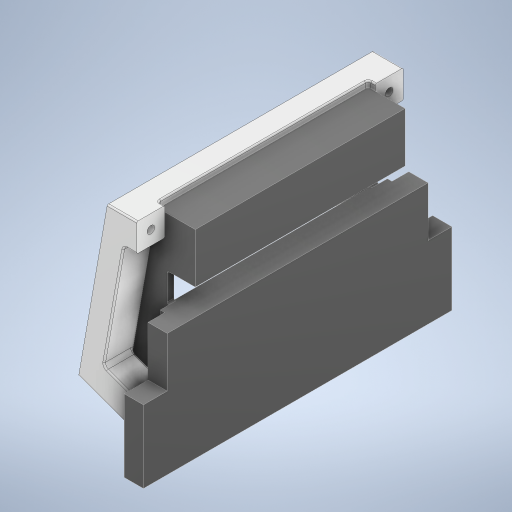
# Autodesk Inventor part: Display Cover
Saved by Autodesk Inventor 2024 (Build 280153000, 153)
## iProperties
Created: 2024-10-16
Part Number: Display Cover
Material: ABS Plastic
Document SubType Name: Modeling
Designer: Ishaan
Density: 1.06 g/cm^3
Appearance: Smooth - White
Author: Ishaan
Autodesk Inventor part; units mm, degrees
sketch "Sketch1" plane through (0, 0, 0) normal (0, 0, 1) x (1, 0, 0)
  line L0 (10.2452, 58.1037) -> (-10.2452, -58.1037)
  line L1 (-10.2452, -58.1037) -> (34.2452, -74.2969)
  line L2 (34.2452, -74.2969) -> (34.2452, -53.0133)
  line L3 (34.2452, -53.0133) -> (7.5941, -43.3131)
  line L4 (7.5941, -43.3131) -> (21.9501, 38.1037)
  line L5 (21.9501, 38.1037) -> (26.2452, 38.1037)
  line L6 (26.2452, 38.1037) -> (26.2452, 58.1037)
  line L7 (26.2452, 58.1037) -> (10.2452, 58.1037)
  point P0 (0, 0)
  point P1 (0, 0)
  dimension "d6" = 118
  dimension "d7" = 20
  dimension "d8" = 15
  dimension "d9" = 100
  dimension "d10" = 100
  dimension "d11" = 20
  dimension "d12" = 16
  dimension "d45" = 8
  constraints: 16 end point, 2 parallel, 2 perpendicular, 1 coincident, 1 horizontal, 1 midpoint, 1 vertical
  measures "d6" distance of L0.start L0.end
  measures "d7" distance of L5.end L6.end
  measures "d8" distance between parallel lines of L0 L4
  measures "d9" angle of L0 L7
  measures "d10" angle of L0 L1
  measures "d11" distance between parallel lines of L1 L3
  measures "d12" distance of L6.end L0.start
  measures "d45" distance between parallel lines of L6 L2
extrude "Extrusion1" add sketch "Sketch1" along normal mid plane 190
ref_plane "Work Plane1" through (1.5725, -60.1874, -95) normal (-0.9848078, 0.1736482, 0) x (0, 0, 1)
sketch "Sketch2" plane through (-10.2452, -58.1037, -95) normal (-0.9848078, 0.1736482, 0) x (0, 0, 1)
  line L0 (190, 0) -> (0, 0) projected
  line L1 (190, 118) -> (190, 0) projected
  line L2 (0, 118) -> (190, 118) projected
  line L3 (0, 0) -> (0, 118) projected
  line L4 (188, 116) -> (188, 2)
  line L5 (188, 2) -> (2, 2)
  line L6 (2, 2) -> (2, 116)
  line L7 (2, 116) -> (188, 116)
  point P0 (95, 59)
  dimension "d16" = 2
  constraints: 8 end point, 3 other
  measures "d16" distance between parallel lines of L2 L7
extrude "Extrusion2" cut sketch "Sketch2" against normal up to surface (12 mm away) contours L4 L5 L6 L7
sketch "Sketch3" plane through (26.2452, 38.1037, 95) normal (1, 0, 0) x (0, 0, -1)
  line L0 (190, 20) -> (0, 20) projected
  line L1 (0, 0) -> (0, 20) projected
  line L2 (190, 0) -> (0, 0) projected
  line L3 (190, 20) -> (190, 0) projected
  line L4 (0, 20) -> (20, 20)
  line L5 (20, 20) -> (20, 0)
  line L6 (20, 0) -> (0, 0)
  line L7 (0, 0) -> (0, 20)
  line L8 (190, 20) -> (170, 20)
  line L9 (170, 20) -> (170, 0)
  line L10 (170, 0) -> (190, 0)
  line L11 (190, 0) -> (190, 20)
  point P0 (95, -38.1037)
  point P1 (170, 20)
  point P2 (20, 20)
  dimension "d19" = 20
  dimension "d20" = 20
  constraints: 16 end point, 4 parallel, 2 horizontal, 2 perpendicular, 2 point on line
  measures "d19" distance of L5.end L6.end
  measures "d20" distance between parallel lines of L3 L9
extrude "Extrusion3" add sketch "Sketch3" along normal blind 5 contours L3 L2 L9 L0 | L5 L2 L1 L0
sketch "Sketch4" plane through (34.2452, -74.2969, -95) normal (-0.3420201, -0.9396926, 0) x (0.9396926, -0.3420201, 0)
  line L0 (0, 0) -> (0, 190) projected
  line L1 (-47.3458, 190) -> (0, 190) projected
  line L2 (-47.3458, 190) -> (-47.3458, 0) projected
  line L3 (0, 0) -> (-47.3458, 0) projected
  line L4 (0, 20) -> (-31.3458, 20)
  line L5 (-31.3458, 20) -> (-31.3458, 170)
  line L6 (-31.3458, 170) -> (0, 170)
  line L7 (0, 170) -> (0, 20)
  line L8 (-45.9608, 20) -> (-41.2623, 20) construction
  line L9 (-45.9608, 170) -> (-41.2623, 170) construction
  point P0 (-57.591, 95)
  point P1 (0, 170)
  dimension "d25" = 16
  constraints: 8 end point, 2 collinear, 2 parallel, 1 horizontal, 1 perpendicular, 1 point on line
  measures "d25" distance between parallel lines of L2 L5
extrude "Extrusion4" cut sketch "Sketch4" against normal blind 1 contours L4 L5 L6 L0
ref_plane "Work Plane2" through (34.2452, -74.2969, 95) normal (0.9396926, -0.3420201, 0) x (0.3420201, 0.9396926, 0)
sketch "Sketch9" plane through (0, 0, 0) normal (0, 0, 1) x (1, 0, 0)
  line L0 (21.7156, 54.0503) -> (9.8979, 56.134) projected
  line L1 (9.8979, 56.134) -> (10.2452, 58.1037) projected
  line L2 (10.2452, 58.1037) -> (26.2452, 58.1037) projected
  line L3 (26.2452, 58.1037) -> (26.2452, 38.1037) projected
  line L4 (26.2452, 38.1037) -> (21.9501, 38.1037) projected
  line L5 (21.9501, 38.1037) -> (7.5941, -43.3131) projected
  line L6 (34.2452, -53.0133) -> (34.2452, -73.2327) projected
  line L7 (34.2452, -73.2327) -> (5.1319, -62.6363) projected
  line L8 (5.1319, -62.6363) -> (4.7898, -63.576) projected
  line L9 (4.7898, -63.576) -> (-10.2452, -58.1037) projected
  line L10 (-10.2452, -58.1037) -> (-9.8979, -56.134) projected
  line L11 (-9.8979, -56.134) -> (1.9197, -58.2178) projected
  line L12 (1.9197, -58.2178) -> (21.7156, 54.0503) projected
  line L13 (21.9501, 38.1037) -> (18.9038, 38.1037)
  line L14 (7.5941, -43.3131) -> (30.2452, -51.5574) construction
  line L15 (21.7156, 54.0503) -> (1.9197, -58.2178) projected
  line L16 (7.5941, -43.3131) -> (34.2452, -53.0133) projected
  line L17 (1.9197, -58.2178) -> (12.9595, -60.1644)
  line L18 (12.9595, -60.1644) -> (34.2452, -67.9118)
  line L19 (7.5941, -43.3131) -> (4.8742, -58.7388)
  point P0 (0, 0)
  dimension "d54" = 5
  constraints: 8 end point, 3 point on line, 2 collinear, 1 horizontal, 1 parallel
  measures "d54" distance between parallel lines of L7 L18
extrude "Extrusion7" cut sketch "Sketch9" along normal mid plane 140 contours L13 L5 L19 L17 L12 | L19 L16 L6 L18 L17
extrude "Extrusion8" cut sketch "Sketch9" along normal up to surface (150 mm away) from surface at -75 contours L19 L16 L6 L18 L17
fillet "Fillet14" radius 1 2 edges at (13.4121, -10.3176, -70) (13.4121, -10.3176, 70)
fillet "Fillet9" radius 1 2 edges at (20.9197, -48.1632, 75) (20.9197, -48.1632, -75)
fillet "Fillet10" radius 3 8 edges at (7.5425, -43.606, -75.2929) (6.146, -51.5259, -75) (7.5941, -43.3131, -85.5) (7.5425, -43.606, 75.2929) (6.146, -51.5259, 75) (7.5941, -43.3131, 85.5) (21.9501, 38.1037, 83) (21.9501, 38.1037, -83)
fillet "Fillet11" radius 10 1 edges at (12.9595, -60.1644, 0)
fillet "Fillet12" radius 2 4 edges at (26.2452, 48.1037, 75) (26.2452, 48.1037, -75) (4.9612, -63.1052, -75) (4.9612, -63.1052, 75)
fillet "Fillet13" radius 1 28 edges at (26.2452, 38.1037, 0) (26.831, 38.1037, -74.4142) (29.7452, 38.1037, -75) (29.7452, 38.1037, 75) (26.831, 38.1037, 74.4142) (26.831, 58.1037, 74.4142) (29.7452, 58.1037, 75) (26.831, 58.1037, -74.4142) (29.7452, 58.1037, -75) (26.2452, 58.1037, 0) (20.7452, 58.1037, -95) (20.7452, 58.1037, 95) (8.3876, -42.855, 95) (14.7721, -2.6047, 95) (27.8563, 38.1037, 95) (22.1024, -48.5937, 95) (8.3876, -42.855, -95) (22.1024, -48.5937, -95) (22.539, 37.4018, -95) (27.8563, 38.1037, -95) (14.7721, -2.6047, -95) (12, -66.2003, -95) (5.3403, -63.7763, -74.4142) (4.7898, -63.576, 0) (5.3403, -63.7763, 74.4142) (20.4572, -69.2784, 75) (20.4572, -69.2784, -75) (12, -66.2003, 95)
fillet "Fillet16" radius 1 3 edges at (10.1473, -11.5571, -70) (18.9038, 38.1037, 0) (10.1473, -11.5571, 70)
sketch "Sketch12" plane through (31.2452, 38.1037, 95) normal (1, 0, 0) x (0, 0, -1)
  line L0 (19, 20) -> (1, 20) projected
  line L1 (189, 20) -> (171, 20) projected
  line L2 (190, 1) -> (190, 19) projected
  point P0 (95, -38.1037)
  point P1 (10, 10)
  point P2 (180, 10)
  point P3 (10, 20)
  point P4 (180, 20)
  point P5 (190, 10)
  constraints: 3 midpoint, 2 horizontal alignment, 2 vertical alignment
hole "Hole4" at (31.2452, 48.1037, 85) at (31.2452, 48.1037, -85) direction (-1, 0, 0) diameter 5.4 end through all
ref_plane "Work Plane3" through (26.2452, 38.1037, 95) normal (1, 0, 0) x (0, 0, -1)
sketch "Sketch13" plane through (26.2452, 38.1037, 95) normal (1, 0, 0) x (0, 0, -1)
  circle A0 centre (10, 10) radius 2.7 projected
  circle A1 centre (10, 10) radius 2.7 projected
  circle A2 centre (180, 10) radius 2.7 projected
  circle A3 centre (180, 10) radius 2.7 projected
  point P0 (95, -38.1037)
hole "Hole5" at (26.2452, 48.1037, -85) at (26.2452, 48.1037, 85) direction (-1, 0, 0) diameter 9.5 end through all
sketch "Sketch14" plane through (0, 0, 0) normal (0, 0, 1) x (1, 0, 0)
  line L0 (9.8979, 56.134) -> (10.2452, 58.1037) projected
  line L1 (10.2452, 58.1037) -> (25.2452, 58.1037) projected
  arc A0 (26.2452, 57.1037) -> (25.2452, 58.1037) centre (25.2452, 57.1037) ccw projected
  line L2 (26.2452, 57.1037) -> (26.2452, 39.1037) projected
  arc A1 (25.2452, 38.1037) -> (26.2452, 39.1037) centre (25.2452, 39.1037) ccw projected
  line L3 (25.2452, 38.1037) -> (20.0956, 38.1037) projected
  arc A2 (19.1108, 39.2773) -> (20.0956, 38.1037) centre (20.0956, 39.1037) ccw projected
  line L4 (19.1108, 39.2773) -> (21.7156, 54.0503) projected
  line L5 (21.7156, 54.0503) -> (9.8979, 56.134) projected
  arc A3 (13.7816, -60.4637) -> (12.0979, -60.0125) centre (10.3614, -69.8606) ccw projected
  line L6 (13.7816, -60.4637) -> (34.2452, -67.9118) projected
  line L7 (34.2452, -67.9118) -> (34.2452, -73.2327) projected
  line L8 (34.2452, -73.2327) -> (5.1319, -62.6363) projected
  arc A4 (3.8501, -63.234) -> (5.1319, -62.6363) centre (4.1922, -62.2943) ccw projected
  line L9 (3.8501, -63.234) -> (-10.2452, -58.1037) projected
  line L10 (-10.2452, -58.1037) -> (-9.8979, -56.134) projected
  line L11 (-9.8979, -56.134) -> (12.0979, -60.0125) projected
  line L12 (52.9452, -1.8963) -> (32.9452, -1.8963) construction
  line L13 (32.9452, -1.8963) -> (32.9452, 18.1037) construction
  line L14 (32.9452, 18.1037) -> (52.9452, 18.1037) construction
  line L15 (52.9452, 18.1037) -> (52.9452, -1.8963) construction
  line L16 (52.9452, -1.8963) -> (32.9452, 18.1037) construction
  line L17 (32.9452, -1.8963) -> (52.9452, 18.1037) construction
  line L18 (52.9452, -1.8963) -> (72.9452, -1.8963) construction
  line L19 (72.9452, -1.8963) -> (72.9452, 53.8537) construction
  line L20 (72.9452, 53.8537) -> (52.9452, 53.8537) construction
  line L21 (52.9452, 53.8537) -> (52.9452, -1.8963) construction
  line L22 (31.2452, 58.1037) -> (28.2452, 58.1037) construction
  line L23 (31.2452, 57.1037) -> (31.2452, 39.1037) construction
  line L24 (52.7452, 53.8537) -> (52.7452, 18.3037)
  line L25 (52.7452, 18.3037) -> (32.7452, 18.3037)
  line L26 (32.7452, -2.0963) -> (50.9452, -2.0963)
  line L27 (50.9452, -2.0963) -> (50.9452, -89.3802)
  line L28 (50.9452, -89.3802) -> (33.9452, -89.3802)
  line L29 (33.9452, -89.3802) -> (33.9452, -52.4785)
  line L30 (33.9452, -52.4785) -> (8.0463, -43.052)
  line L31 (8.0463, -43.052) -> (22.2857, 37.7037)
  line L32 (22.2857, 37.7037) -> (26.6452, 37.7037)
  line L33 (26.6452, 37.7037) -> (26.6452, 53.8537)
  line L34 (26.6452, 53.8537) -> (52.7452, 53.8537)
  line L35 (32.7452, 18.3037) -> (32.7452, -2.0963)
  line L36 (34.2452, -53.0133) -> (9.9596, -44.1741) projected
  arc A5 (8.0313, -40.834) -> (9.9596, -44.1741) centre (10.9857, -41.355) ccw projected
  line L37 (4.8742, -58.7388) -> (21.513, 35.6246) projected
  circle A6 centre (10.9857, -41.355) radius 2.6
  line L38 (28.2452, 38.1037) -> (31.2452, 38.1037) projected
  arc A7 (24.4674, 38.1037) -> (21.513, 35.6246) centre (24.4674, 35.1037) ccw projected
  circle A8 centre (24.4674, 35.1037) radius 2.6
  line L39 (26.6452, 37.7037) -> (52.7452, 37.7037)
  line L40 (33.9452, -89.3802) -> (37.1952, -89.3802)
  line L41 (37.1952, -89.3802) -> (37.1952, -77.3802)
  line L42 (37.1952, -77.3802) -> (33.9452, -77.3802)
  line L43 (33.9452, -77.3802) -> (33.9452, -89.3802)
  line L44 (-10.2452, -58.1037) -> (34.2452, -74.2969) construction
  line L45 (33.9452, -77.3802) -> (23.2544, -73.4891) construction
  line L46 (33.9452, -67.3769) -> (5.5778, -57.052)
  line L47 (5.5778, -57.052) -> (8.0463, -43.052)
  line L48 (33.9452, -52.4785) -> (47.9452, -57.574)
  line L49 (47.9452, -57.574) -> (47.9452, 37.7037)
  line L50 (32.7452, -2.0963) -> (47.9452, -2.0963)
  line L51 (47.9452, -2.0963) -> (47.9452, -9.0963)
  line L52 (47.9452, -9.0963) -> (32.7452, -9.0963)
  line L53 (32.7452, -9.0963) -> (32.7452, -2.0963)
  line L54 (33.9452, -67.3769) -> (47.9452, -72.4725)
  line L55 (47.9452, -72.4725) -> (47.9452, -57.574)
  point P0 (0, 0)
  point P1 (42.9452, 8.1037)
  point P2 (24.4674, 37.7037)
  point P3 (21.9069, 35.5551)
  point P4 (8.4252, -40.9035)
  point P5 (10.0964, -43.7982)
  point P6 (10.0964, -43.7982)
  point P7 (47.9452, 18.3037)
  dimension "d98" = 20
  dimension "d99" = 20
  dimension "d100" = 4.25
  dimension "d101" = 45.75
  dimension "d102" = 20
  dimension "d104" = 21.7
  dimension "d105" = 32.9452
  dimension "d106" = 0.2
  dimension "d107" = 0.4
  dimension "d108" = 0.2
  dimension "d109" = 0.2
  dimension "d110" = 1
  dimension "d111" = 0.2
  dimension "d112" = 0.4
  dimension "d113" = 0.4
  dimension "d114" = 0.4
  dimension "d115" = 8
  dimension "d116" = 3.25
  dimension "d117" = 12
  dimension "d118" = 3
  dimension "d142" = 0.4
  dimension "d146" = 3
  dimension "d147" = 7
  constraints: 76 end point, 14 parallel, 10 perpendicular, 5 collinear, 4 horizontal, 4 point on line, 2 centre point, 2 coincident, 2 midpoint, 2 tangent, 1 vertical
  measures "d98" distance of L13.end L14.end
  measures "d99" distance of L12.end L13.end
  measures "d100" distance between parallel lines of L20 L22
  measures "d101" distance from line of L20 point (42.945, 8.104)
  measures "d102" distance between parallel lines of L19 L21
  measures "d104" distance between parallel lines of L21 L23
  measures "d105" distance from line of point (0, 0) L13
  measures "d106" distance between parallel lines of L21 L24
  measures "d107" distance between parallel lines of L33 L2
  measures "d108" distance between parallel lines of L25 L14
  measures "d109" distance between parallel lines of L12 L26
  measures "d110" distance between parallel lines of L29 L13
  measures "d111" distance between parallel lines of L13 L35
  measures "d112" distance between parallel lines of L30 L36
  measures "d113" distance between parallel lines of L37 L31
  measures "d114" distance between parallel lines of L38 L32
  measures "d115" distance from line of L27 point (42.945, 8.104)
  measures "d116" distance between parallel lines of L29 L41
  measures "d117" distance of L40.end L41.end
  measures "d118" distance between parallel lines of L44 L45
  measures "d142" distance between parallel lines of L46 L6
  measures "d146" distance between parallel lines of L27 L49
  measures "d147" distance between parallel lines of L26 L52
ref_plane "Work Plane4" through (0, 0, 98) normal (0, 0, 1) x (1, 0, 0)
ref_plane "Work Plane5" through (0, 0, -98) normal (0, 0, -1) x (-1, 0, 0)
extrude "Extrusion9" add sketch "Sketch14" along normal up to surface (196 mm away) from surface at -98 separate body contours L29 L54 L55 L49 L26 L27 L28 L41 L42 L8 L7 L6 | L6 L7 L8 L29 | L29 L48 L55 L54 | L30 A6 L31 A8 L32 L39 L49 L25 L35 L53 L52 L48 | A6 | L52 L53 L26 L49 | A8 | L49 L39 L24 L25
sketch "Sketch15" plane through (24.4674, 37.7037, 98) normal (0, 1, 0) x (1, 0, 0)
  line L0 (6.7778, 23) -> (3.7778, 23) projected
  arc A0 (1.7778, 25) -> (3.7778, 23) centre (3.7778, 25) ccw projected
  line L1 (1.7778, 25) -> (1.7778, 171) projected
  arc A1 (3.7778, 173) -> (1.7778, 171) centre (3.7778, 171) ccw projected
  line L2 (3.7778, 173) -> (6.7778, 173) projected
  line L3 (28.2778, 23.2) -> (3.7778, 23.2)
  arc A2 (1.9778, 25) -> (3.7778, 23.2) centre (3.7778, 25) ccw
  line L4 (1.9778, 25) -> (1.9778, 171)
  arc A3 (3.7778, 172.8) -> (1.9778, 171) centre (3.7778, 171) ccw
  line L5 (3.7778, 172.8) -> (28.2778, 172.8)
  line L6 (28.2778, 196) -> (28.2778, 0) projected
  point P0 (-24.4674, 98)
  dimension "d123" = 0.2
  constraints: 6 end point, 4 point on circle, 2 centre point, 2 point on line, 4 other
  measures "d123" radial gap between concentric circles of A1 A3
ref_plane "Work Plane6" through (10.2452, 53.8537, 94) normal (0, 1, 0) x (1, 0, 0)
extrude "Extrusion10" add sketch "Sketch15" along normal up to surface (16.15 mm away) bodies 2
sketch "Sketch16" plane through (24.4674, 37.7037, 98) normal (0, 0, 1) x (1, 0, 0)
  arc A0 (0, 0) -> (-2.5605, -2.1485) centre (0, -2.6) ccw projected
  line L0 (-16.0422, -78.6072) -> (-2.5605, -2.1485) projected
  arc A1 (-16.0422, -78.6072) -> (-14.371, -81.5019) centre (-13.4817, -79.0586) ccw projected
  line L1 (9.4778, -90.1821) -> (-14.371, -81.5019) projected
  line L2 (9.4778, -115.0839) -> (9.4778, -90.1821) projected
  line L3 (12.7278, -115.0839) -> (9.4778, -115.0839) projected
  line L4 (12.7278, -127.0839) -> (12.7278, -115.0839) projected
  line L5 (26.4778, -127.0839) -> (12.7278, -127.0839) projected
  line L6 (26.4778, -39.8) -> (26.4778, -127.0839) projected
  line L7 (8.2778, -39.8) -> (26.4778, -39.8) projected
  line L8 (8.2778, -19.4) -> (8.2778, -39.8) projected
  line L9 (28.2778, -19.4) -> (8.2778, -19.4) projected
  line L10 (28.2778, 0) -> (28.2778, -19.4) projected
  line L11 (0, 0) -> (28.2778, 0) projected
  line L12 (9.4778, -90.1821) -> (9.4778, -39.8)
  line L13 (9.4778, -90.1821) -> (-14.371, -81.5019) projected
  line L14 (9.7778, -90.717) -> (-14.5078, -81.8777) projected
  line L15 (9.4778, -87.4152) -> (26.4778, -87.4152)
  dimension "d131" = 3
  constraints: 4 end point, 3 point on line, 2 perpendicular
  measures "d131" distance from line of L15.start L14
extrude "Extrusion11" cut sketch "Sketch16" against normal up to surface (23.2 mm away) contours L11 L10 L9 L8 L7 L12 L1 A1 L0 A0 | L12 L7 L6 L15 bodies 2
mirror "Mirror1" about plane through (0, 0, 0) normal (0, 0, 1) of "Extrusion11" bodies 2
fillet "Fillet17" radius 1.2 2 edges at (32.7452, 18.3037, 0) (32.7452, -2.0963, 0)
sketch "Sketch17" plane through (50.9452, -89.3802, 98) normal (1, 0, 0) x (0, 0, -1)
  line L0 (172.8, 39.6686) -> (172.8, 87.2839) projected
  line L1 (172.8, 87.2839) -> (23.2, 87.2839) projected
  line L2 (23.2, 87.2839) -> (23.2, 39.6686) projected
  line L3 (23.2, 39.6686) -> (0, 39.6686) projected
  line L4 (0, 39.6686) -> (0, 0) projected
  line L5 (196, 0) -> (0, 0) projected
  line L6 (196, 0) -> (196, 39.6686) projected
  line L7 (196, 39.6686) -> (172.8, 39.6686) projected
  line L8 (17, 87.2839) -> (179, 87.2839)
  line L9 (179, 87.2839) -> (179, 39.6686)
  line L10 (179, 39.6686) -> (17, 39.6686)
  line L11 (17, 39.6686) -> (17, 87.2839)
  line L12 (23, 35.3027) -> (23, 44.0252) projected
  line L13 (173, 44.0252) -> (173, 35.3027) projected
  point P0 (98, 89.3802)
  point P1 (17, 39.6686)
  point P2 (23.2, 39.6686)
  point P3 (172.8, 39.6686)
  point P4 (179, 39.6686)
  point P5 (172.8, 87.2839)
  point P6 (23.2, 87.2839)
  dimension "d132" = 6
  dimension "d133" = 6
  constraints: 8 end point, 2 collinear, 2 parallel, 1 horizontal, 1 perpendicular
  measures "d132" distance between parallel lines of L11 L12
  measures "d133" distance between parallel lines of L9 L13
extrude "Extrusion12" add sketch "Sketch17" against normal up to surface (17 mm away) contours L10 L2 L1 L0 | L0 L8 L9 L7 | L3 L11 L8 L2 bodies 2
sketch "Sketch18" plane through (50.9452, -89.3802, 98) normal (1, 0, 0) x (0, 0, -1)
  line L0 (17, 39.6686) -> (0, 39.6686) projected
  line L1 (0, 39.6686) -> (0, 0) projected
  line L2 (196, 0) -> (0, 0) projected
  line L3 (196, 0) -> (196, 39.6686) projected
  line L4 (196, 39.6686) -> (179, 39.6686) projected
  line L5 (179, 39.6686) -> (179, 87.2839) projected
  line L6 (179, 87.2839) -> (17, 87.2839) projected
  line L7 (17, 87.2839) -> (17, 39.6686) projected
  line L8 (0, 0) -> (0, 12) projected
  line L9 (196, 12) -> (0, 12) projected
  line L10 (196, 12) -> (196, 0) projected
  line L11 (196, 0) -> (0, 0) projected
  line L12 (0, 0) -> (-12, 0)
  line L13 (-12, 0) -> (-12, 51.6686)
  line L14 (-12, 51.6686) -> (0, 51.6686)
  line L15 (0, 51.6686) -> (0, 0)
  line L16 (0, 51.6686) -> (17, 51.6686)
  line L17 (17, 51.6686) -> (17, 39.6686)
  line L18 (17, 39.6686) -> (0, 39.6686)
  line L19 (0, 39.6686) -> (0, 51.6686)
  line L20 (17, 87.2839) -> (5, 87.2839)
  line L21 (5, 87.2839) -> (5, 51.6686)
  line L22 (5, 51.6686) -> (17, 51.6686)
  line L23 (17, 51.6686) -> (17, 87.2839)
  point P0 (98, 89.3802)
  dimension "d136" = 12
  dimension "d137" = 12
  dimension "d138" = 12
  dimension "d139" = 12
  constraints: 24 end point, 6 parallel, 3 horizontal, 3 perpendicular, 1 point on line
  measures "d136" distance between parallel lines of L2 L9
  measures "d137" distance between parallel lines of L1 L13
  measures "d138" distance between parallel lines of L7 L21
  measures "d139" distance between parallel lines of L0 L16
extrude "Extrusion13" add sketch "Sketch18" against normal up to surface (13.75 mm away) contours L0 L15 L16 L7 | L1 L12 L13 L14 L15 | L16 L21 L20 L7 bodies 2
mirror "Mirror2" about plane through (0, 0, 0) normal (0, 0, 1) of "Extrusion13" bodies 2
extrude "Extrusion14" add sketch "Sketch14" along normal up to surface (149.6 mm away) from surface at -74.8 contours L46 L47 L30 A5 L36 L29 | L36 A5 L30 L29 | A5 L30 L31 | L31 A6 L30 A5 bodies 2
fillet "Fillet18" radius 2 1 edges at (5.5778, -57.052, 0)
extrude "Extrusion15" cut sketch "Sketch14" along normal mid plane 140 contours L46 L47 L30 A5 L36 L29 | L29 L48 L55 L54 | L36 A5 L30 L29 | A5 L30 L31 | L31 A6 L30 A5 | L30 A6 L31 A8 L32 L39 L49 L25 L35 L53 L52 L48 | A6 | A8 bodies 2
sketch "Sketch19" plane through (52.7452, 18.3037, -74.8) normal (1, 0, 0) x (0, 0, -1)
  line L0 (0, 0) -> (-149.6, 0) projected
  line L1 (18.2, -20.4) -> (-167.8, -20.4) projected
  line L2 (-144.8, -19.2) -> (-144.8, -1.2) projected
  line L3 (-4.8, -1.2) -> (-4.8, -19.2) projected
  line L4 (-144.8, 0) -> (-4.8, 0)
  line L5 (-4.8, 0) -> (-4.8, -20.4)
  line L6 (-4.8, -20.4) -> (-144.8, -20.4)
  line L7 (-144.8, -20.4) -> (-144.8, 0)
  point P0 (-74.8, -18.3037)
  constraints: 8 end point, 4 collinear, 2 parallel, 1 horizontal, 1 perpendicular
extrude "Extrusion16" cut sketch "Sketch19" against normal through all bodies 2
sketch "Sketch10" plane through (1.9197, -58.2178, -93) normal (-0.9848078, 0.1736482, 0) x (0, 0, 1)
  line L0 (0, 114) -> (186, 114) construction
  line L1 (0, 114) -> (186, 0) construction
  line L2 (0, 0) -> (0, 114) construction
  line L3 (0, 0) -> (186, 114) construction
  line L4 (172.6, 7.66) -> (17.7, 7.66)
  line L5 (17.7, 7.66) -> (17.7, 99.66)
  line L6 (17.7, 99.66) -> (172.6, 99.66)
  line L7 (172.6, 99.66) -> (172.6, 7.66)
  line L8 (172.6, 7.66) -> (17.7, 99.66) construction
  line L9 (17.7, 7.66) -> (172.6, 99.66) construction
  point P0 (95.15, 53.66)
  point P1 (93, 57)
  point P2 (93, 57)
  dimension "d48" = 154.9
  dimension "d49" = 92
  dimension "d50" = 3.34
  dimension "d51" = 2.15
  constraints: 16 end point, 4 coincident, 4 midpoint, 2 parallel, 1 horizontal, 1 perpendicular
  measures "d48" distance of L5.end L6.end
  measures "d49" distance of L4.end L5.end
  measures "d50" vertical distance of point (95.15, 53.66) point (93, 57)
  measures "d51" horizontal distance of point (93, 57) point (95.15, 53.66)
sketch "Sketch11" plane through (7.5941, -43.3131, -75) normal (0.9848078, -0.1736482, 0) x (0, 0, -1)
  point P0 (-75, 41.3364)
  point P1 (0.3, 83.9964)
  point P2 (-154.6, 83.9964)
  point P3 (-154.6, -8.0036)
  point P4 (0.3, -8.0036)
equation "\"d10\" = d9"
equation "\"d11\" = d7"
equation "\"d20\" = d19"
equation "\"d25\" = d12"
equation "\"d109\" = d108"
equation "\"d111\" = d108"
equation "\"d113\" = d112"
equation "\"d114\" = d113"
body "Solid1"
